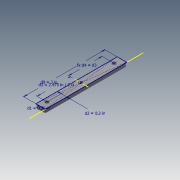
# Autodesk Inventor part: Standard
Saved by Autodesk Inventor 2020.3 (Build 243373000, 373)
## iProperties
RuleStatus: InUse
AfterDocSave0: file://Part Number Cleaner
Created: 2023-02-10
Material: Generic
Catalog Web Link: https://www.janelia.org/
Vendor: HHMI: JRC - jET
Document SubType Name: Modeling
Designer: arnoldj
Density: 1 g/cm^3
Appearance: Default
DESIGN DEPARTMENT: HHMI: JRC - jET
ALTERED ITEM PART NUMBER: N/A
ALTERED ITEM VENDOR: N/A
ALTERED ITEM DESCRIPTION: N/A
Title: Standard
Author: arnoldj
Revision Number: 0
Autodesk Inventor part; units mm, degrees
ref_plane "YZ Plane" through (0, 0, 0) normal (1, 0, 0) x (0, 1, 0)
ref_plane "XZ Plane" through (0, 0, 0) normal (0, 1, 0) x (-1, 0, 0)
ref_plane "XY Plane" through (0, 0, 0) normal (0, 0, 1) x (1, 0, 0)
sketch "Sketch1" plane through (0, 0, 0) normal (0, 1, 0) x (-1, 0, 0)
  line L0 (-1.778, 0) -> (10.668, 0) projected
  line L1 (0, -53.34) -> (0, 53.34) projected
  line L2 (8.89, -38.1) -> (0, -38.1)
  line L3 (0, -38.1) -> (0, 38.1)
  line L4 (0, 38.1) -> (8.89, 38.1)
  line L5 (8.89, 38.1) -> (8.89, -38.1)
  line L6 (8.89, -38.1) -> (0, 38.1) construction
  line L7 (0, -38.1) -> (8.89, 38.1) construction
  point P0 (0, 0)
  point P1 (4.445, 0)
  point P2 (5.08, 31.4325)
  point P3 (5.08, 0)
  point P4 (5.08, -31.4325)
  dimension "d0" = 76.2
  dimension "d1" = 8.89
  dimension "d2" = 5.08
  dimension "d3" = 31.4325
  dimension "d4" = 31.4325
  constraints: 12 end point, 3 midpoint, 2 parallel, 2 point on line, 2 vertical alignment, 1 horizontal, 1 perpendicular
  measures "d0" distance of L4.end L2.start
  measures "d1" distance of L3.end L4.end
  measures "d2" distance from line of point (5.08, 31.433) L3
  measures "d3" distance from line of L0 point (5.08, 31.433)
  measures "d4" distance from line of point (5.08, -31.433) L0
extrude "Extrusion1" add sketch "Sketch1" against normal blind 3.175
fillet "Fillet1" radius 1.27 2 edges at (-8.89, -1.5875, 38.1) (-8.89, -1.5875, -38.1)
fillet "Fillet2" radius 1.27 2 edges at (0, -1.5875, 38.1) (0, -1.5875, -38.1)
hole "Hole1" at (-5.08, 0, 31.4325) at (-5.08, 0, 0) at (-5.08, 0, -31.4325) direction (0, -1, 0) diameter 2.9972 end through all
equation "\"d4\" = d3"
body "Solid1"
